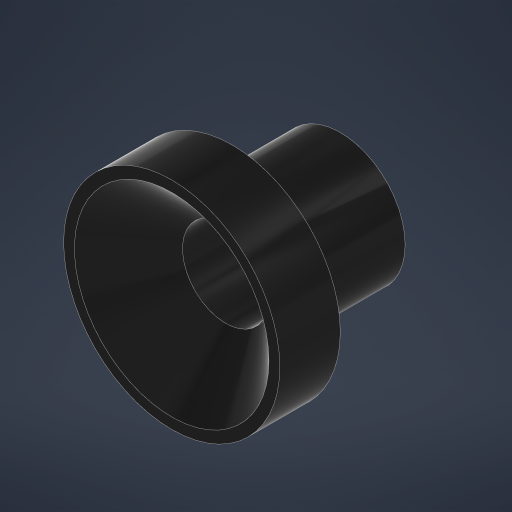
# Autodesk Inventor part: Handmade tiered cover
Saved by Autodesk Inventor 2024 (Build 280153000, 153)
## iProperties
Created: 2024-01-24
Part Number: Handmade tiered cover
Material: LCP 플라스틱
Document SubType Name: Modeling
Designer: ASUS
Density: 1.626 g/cm^3
Appearance: 매끄러움 - 검은색
Author: ASUS
Autodesk Inventor part; units mm, degrees
ref_plane "YZ Plane" through (0, 0, 0) normal (1, 0, 0) x (0, 1, 0)
sketch "스케치1" plane through (0, 0, 0) normal (0, 0, 1) x (1, 0, 0)
  line L0 (5, 1.4434) -> (6.25, 0.7217) projected
  line L1 (6.25, 0.7217) -> (6.25, -0.7217) projected
  line L2 (6.25, -0.7217) -> (5, -1.4434) projected
  line L3 (5, -1.4434) -> (3.75, -0.7217) projected
  line L4 (3.75, -0.7217) -> (3.75, 0.7217) projected
  line L5 (3.75, 0.7217) -> (5, 1.4434) projected
  circle A0 centre (5, 0) radius 5 projected
  circle A1 centre (5, 0) radius 5
  point P0 (0, 0)
  constraints: 1 centre point, 1 coincident, 1 horizontal alignment, 1 other
ref_plane "작업 평면1" through (-0.2823, -5.2823, -2.8) normal (0, 0, -1) x (0, 1, 0)
extrude "돌출1" add sketch "스케치1" against normal up to surface (2.8 mm away)
sketch "스케치2" plane through (5, 0, -2.8) normal (0, 0, -1) x (-1, 0, 0)
  circle A0 centre (0, 0) radius 3 projected
  circle A1 centre (0, 0) radius 2 projected
  point P0 (5, 0)
ref_plane "작업 평면2" through (1.8306, -3.1694, -7.8) normal (0, 0, -1) x (0, 1, 0)
extrude "돌출2" add sketch "스케치2" along normal up to surface (5 mm away)
sketch "스케치3" plane through (5, 0, 0) normal (0, 0, 1) x (1, 0, 0)
  circle A0 centre (0, 0) radius 5 projected
  line L0 (0, 1.4434) -> (1.25, 0.7217) projected
  line L1 (1.25, 0.7217) -> (1.25, -0.7217) projected
  line L2 (1.25, -0.7217) -> (0, -1.4434) projected
  line L3 (0, -1.4434) -> (-1.25, -0.7217) projected
  line L4 (-1.25, -0.7217) -> (-1.25, 0.7217) projected
  line L5 (-1.25, 0.7217) -> (0, 1.4434) projected
  circle A1 centre (0, 0) radius 2
  point P0 (-5, 0)
  dimension "d4" = 4
  constraints: 1 centre point, 1 coincident
  measures "d4" diameter of A1
extrude "돌출3" cut sketch "스케치3" against normal through all contours L0 L1 L2 L3 L4 L5 | A1
chamfer "모따기1" distance 2.5 angle 45 1 edges at (3, 0, 0)
